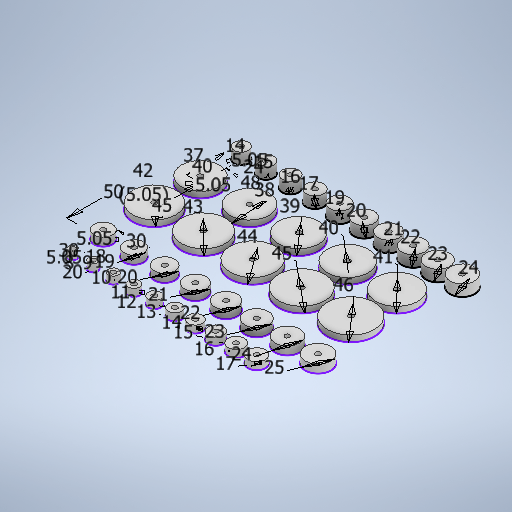
# Autodesk Inventor part: shinrotationblock
Saved by Autodesk Inventor 2025.2 (Build 292293000, 293)
## iProperties
Created: 2025-01-15
Part Number: shinrotationblock
Material: Generic
Document SubType Name: Modeling
Designer: email
Density: 1 g/cm^3
Appearance: Default
Author: email
Autodesk Inventor part; units mm, degrees
ref_plane "YZ Plane" through (0, 0, 0) normal (1, 0, 0) x (0, 1, 0)
ref_plane "XZ Plane" through (0, 0, 0) normal (0, 1, 0) x (-1, 0, 0)
ref_plane "XY Plane" through (0, 0, 0) normal (0, 0, 1) x (1, 0, 0)
sketch "Sketch1" plane through (0, 0, 0) normal (0, 1, 0) x (-1, 0, 0)
  circle A0 centre (0, 0) radius 2.525
  line L0 (0, 0) -> (-26.9577, 0) construction
  circle A1 centre (-24, 0) radius 2.525
  circle A2 centre (-48, 0) radius 2.525
  circle A3 centre (-72, 0) radius 2.525
  circle A4 centre (-96, 0) radius 2.525
  circle A5 centre (-120, 0) radius 2.525
  circle A6 centre (-144, 0) radius 2.525
  circle A7 centre (-168, 0) radius 2.525
  circle A8 centre (0, 0) radius 7
  circle A9 centre (-24, 0) radius 7.5
  circle A10 centre (-48, 0) radius 8
  circle A11 centre (-72, 0) radius 8.5
  circle A12 centre (-96, 0) radius 9.5
  circle A13 centre (-120, 0) radius 10
  circle A14 centre (-144, 0) radius 10.5
  circle A15 centre (-168, 0) radius 11
  circle A16 centre (-192, 0) radius 2.525
  circle A17 centre (-216, 0) radius 2.525
  circle A18 centre (-192, 0) radius 11.5
  circle A19 centre (-216, 0) radius 12
  circle A20 centre (0, 40) radius 2.525
  circle A21 centre (-48, 40) radius 2.525
  circle A22 centre (-96, 40) radius 2.525
  circle A23 centre (-144, 40) radius 2.525
  circle A24 centre (-192, 40) radius 2.525
  circle A25 centre (0, 40) radius 18.5
  circle A26 centre (-48, 40) radius 19
  circle A27 centre (-96, 40) radius 19.5
  circle A28 centre (-144, 40) radius 20
  circle A29 centre (-192, 40) radius 20.5
  circle A30 centre (0, 135) radius 2.525
  circle A31 centre (-30, 135) radius 2.525
  circle A32 centre (-60, 135) radius 2.525
  circle A33 centre (-90, 135) radius 2.525
  circle A34 centre (-120, 135) radius 2.525
  circle A35 centre (-150, 135) radius 2.525
  circle A36 centre (-180, 135) radius 2.525
  circle A37 centre (-210, 135) radius 2.525
  circle A38 centre (0, 135) radius 9
  circle A39 centre (-30, 135) radius 9.5
  circle A40 centre (-60, 135) radius 10
  circle A41 centre (-90, 135) radius 10.5
  circle A42 centre (-120, 135) radius 11
  circle A43 centre (-150, 135) radius 11.5
  circle A44 centre (-180, 135) radius 12
  circle A45 centre (-210, 135) radius 12.5
  circle A46 centre (0, 165) radius 2.525
  circle A47 centre (-20, 165) radius 2.525
  circle A48 centre (-40, 165) radius 2.525
  circle A49 centre (-60, 165) radius 2.525
  circle A50 centre (-80, 165) radius 2.525
  circle A51 centre (-100, 165) radius 2.525
  circle A52 centre (-120, 165) radius 2.525
  circle A53 centre (-140, 165) radius 2.525
  circle A54 centre (-160, 165) radius 2.525
  circle A55 centre (-180, 165) radius 2.525
  circle A56 centre (0, 165) radius 4
  circle A57 centre (-20, 165) radius 4.5
  circle A58 centre (-40, 165) radius 5
  circle A59 centre (-60, 165) radius 5.5
  circle A60 centre (-80, 165) radius 6
  circle A61 centre (-100, 165) radius 6.5
  circle A62 centre (-120, 165) radius 7
  circle A63 centre (-140, 165) radius 7.5
  circle A64 centre (-160, 165) radius 8
  circle A65 centre (-180, 165) radius 8.5
  line L1 (0, 0) -> (0, 13.0179) construction
  circle A66 centre (0, 85) radius 2.525
  circle A67 centre (-48, 85) radius 2.525
  circle A68 centre (-96, 85) radius 2.525
  circle A69 centre (-144, 85) radius 2.525
  circle A70 centre (-192, 85) radius 2.525
  circle A71 centre (0, 85) radius 21
  circle A72 centre (-48, 85) radius 21.5
  circle A73 centre (-96, 85) radius 22
  circle A74 centre (-144, 85) radius 22.5
  circle A75 centre (-192, 85) radius 23
  dimension "d0" = 5.05
  dimension "d3" = 24
  dimension "d8" = 14
  dimension "d9" = 15
  dimension "d10" = 16
  dimension "d11" = 17
  dimension "d12" = 19
  dimension "d13" = 20
  dimension "d14" = 21
  dimension "d15" = 22
  dimension "d16" = 23
  dimension "d17" = 24
  dimension "d18" = 5.05
  dimension "d19" = 40
  dimension "d22" = 48
  dimension "d27" = 37
  dimension "d28" = 38
  dimension "d29" = 39
  dimension "d30" = 40
  dimension "d31" = 41
  dimension "d38" = 5.05
  dimension "d41" = 30
  dimension "d46" = 18
  dimension "d47" = 19
  dimension "d48" = 20
  dimension "d49" = 21
  dimension "d50" = 22
  dimension "d51" = 23
  dimension "d52" = 24
  dimension "d53" = 25
  dimension "d56" = 30
  dimension "d57" = 5.05
  dimension "d60" = 20
  dimension "d65" = 8
  dimension "d25" = 45
  dimension "d67" = 50
  dimension "d68" = 42
  dimension "d69" = 43
  dimension "d70" = 44
  dimension "d71" = 45
  dimension "d72" = 46
  dimension "d73" = 5.05
  dimension "d74" = 9
  dimension "d75" = 10
  dimension "d76" = 11
  dimension "d77" = 12
  dimension "d78" = 13
  dimension "d79" = 14
  dimension "d80" = 15
  dimension "d81" = 16
  dimension "d82" = 17
  constraints: 76 centre point, 39 coincident, 5 horizontal, 4 end point, 2 vertical, 68 other
  measures "d0" diameter of A0
  measures "d3" distance of L0.start A1.centre
  measures "d8" diameter of A8
  measures "d9" diameter of A9
  measures "d10" diameter of A10
  measures "d11" diameter of A11
  measures "d12" diameter of A12
  measures "d13" diameter of A13
  measures "d14" diameter of A14
  measures "d15" diameter of A15
  measures "d16" diameter of A18
  measures "d17" diameter of A19
  measures "d18" diameter of A20
  measures "d19" distance of A20.centre point (0, 0)
  measures "d22" distance of A20.centre A21.centre
  measures "d27" diameter of A25
  measures "d28" diameter of A26
  measures "d29" diameter of A27
  measures "d30" diameter of A28
  measures "d31" diameter of A29
  measures "d38" diameter of A30
  measures "d41" distance of A30.centre A31.centre
  measures "d46" diameter of A38
  measures "d47" diameter of A39
  measures "d48" diameter of A40
  measures "d49" diameter of A41
  measures "d50" diameter of A42
  measures "d51" diameter of A43
  measures "d52" diameter of A44
  measures "d53" diameter of A45
  measures "d56" distance of A46.centre A30.centre
  measures "d57" diameter of A46
  measures "d60" distance of A46.centre A47.centre
  measures "d65" diameter of A56
  measures "d25" distance of A20.centre A66.centre
  measures "d67" distance of A66.centre A30.centre
  measures "d68" diameter of A71
  measures "d69" diameter of A72
  measures "d70" diameter of A73
  measures "d71" diameter of A74
  measures "d72" diameter of A75
  measures "d73" diameter of A66
  measures "d74" diameter of A57
  measures "d75" diameter of A58
  measures "d76" diameter of A59
  measures "d77" diameter of A60
  measures "d78" diameter of A61
  measures "d79" diameter of A62
  measures "d80" diameter of A63
  measures "d81" diameter of A64
  measures "d82" diameter of A65
extrude "Extrusion1" add sketch "Sketch1" along normal blind 11 contours A8 | A9 | A10 | A11 | A12 | A13 | A14 | A15 | A18 | A19
extrude "Extrusion2" add sketch "Sketch1" along normal blind 6 contours A25 | A26 | A27 | A28 | A29 | A71 | A72 | A73 | A74 | A75
extrude "Extrusion3" add sketch "Sketch1" along normal blind 8 contours A38 | A39 | A40 | A41 | A42 | A43 | A44 | A45
extrude "Extrusion4" add sketch "Sketch1" along normal blind 7.1 contours A56 | A57 | A58 | A59 | A60 | A61 | A62 | A63 | A64 | A65
body "Solid1"
